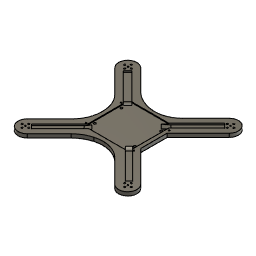
drone frame v1 (Autodesk Fusion 360 design; units mm, degrees)
Autodesk Fusion 360 part; units mm, degrees
note: some values were not read from the file. Chosen so that the rebuilt part matches the saved one: which face or edge a step refers to; which pieces of a blend or face edit are solid. Set by a fixed rule: which sketch regions a step uses.
sketch "Sketch1" plane through (0, 0, 0) normal (0, 1, 0) x (1, 0, 0)
  line L0 (0, 0) -> (-60, 0)
  line L1 (-60, 0) -> (-60, 60)
  line L2 (-60, 60) -> (0, 60)
  line L3 (0, 60) -> (0, 0)
  line L4 (5, -5) -> (-65, -5)
  line L5 (-65, -5) -> (-65, 65)
  line L6 (-65, 65) -> (5, 65)
  line L7 (5, 65) -> (5, -5)
  dimension "d1" = 60
  dimension "d2" = 60
  dimension "d4" = 5
  dimension "d5" = 5
  dimension "d6" = 5
  constraint horizontal L0
  constraint vertical L1
  constraint horizontal L2
  constraint vertical L3
  constraint coincident L0.start L3.end
  constraint horizontal L4
  constraint vertical L5
  constraint horizontal L6
  constraint vertical L7
  measures "d1" distance of L0.start L0.end
  measures "d2" distance of L0.start L2.end
  measures "d4" distance of L0 L4
  measures "d5" distance of L2 L6
  measures "d6" distance of L1 L5
sketch "Sketch2" plane through (0, 0, 0) normal (0, 1, 0) x (1, 0, 0)
  line L0 (-65.6777, 47.3223) -> (-48, 65)
  line L1 (-48, 65) -> (-90.4264, 107.4264)
  line L2 (-108.1041, 89.7487) -> (-65.6777, 47.3223)
  line L3 (-12.6777, 65.6777) -> (5, 48)
  line L4 (5, 48) -> (47.4264, 90.4264)
  line L5 (29.7487, 108.1041) -> (-12.6777, 65.6777)
  line L6 (-47.3223, -5.6777) -> (-65, 12)
  line L7 (-65, 12) -> (-107.4264, -30.4264)
  line L8 (-89.7487, -48.1041) -> (-47.3223, -5.6777)
  line L9 (-12.6777, -5.6777) -> (5, 12)
  line L10 (5, 12) -> (47.4264, -30.4264)
  line L11 (29.7487, -48.1041) -> (-12.6777, -5.6777)
  arc A0 (-90.4264, 107.4264) -> (-108.1041, 89.7487) centre (-99.2652, 98.5876) ccw
  arc A1 (47.4264, 90.4264) -> (29.7487, 108.1041) centre (38.5876, 99.2652) ccw
  arc A2 (29.7487, -48.1041) -> (47.4264, -30.4264) centre (38.5876, -39.2652) ccw
  arc A3 (-107.4264, -30.4264) -> (-89.7487, -48.1041) centre (-98.5876, -39.2652) ccw
  dimension "d7" = 60
  dimension "d8" = 60
  dimension "d9" = 60
  dimension "d10" = 60
  dimension "d11" = 25
  dimension "d12" = 25
  dimension "d13" = 25
  dimension "d14" = 25
  constraint perpendicular L0 L1
  constraint parallel L1 L2
  constraint perpendicular L3 L4
  constraint parallel L4 L5
  constraint perpendicular L6 L7
  constraint parallel L7 L8
  constraint perpendicular L9 L10
  constraint parallel L10 L11
  constraint tangent L2 A0
  constraint tangent L1 A0
  constraint tangent L11 A2
  constraint tangent L10 A2
  constraint tangent L8 A3
  measures "d7" distance of L0.start L2.start
  measures "d8" distance of L3.start L5.start
  measures "d9" distance of L6.start L8.start
  measures "d10" distance of L9.start L11.start
  measures "d11" distance of L7 L8
  measures "d12" distance of L1 L2
  measures "d13" distance of L4 L5
  measures "d14" distance of L10 L11
extrude "Extrude1" add sketch "Sketch1" sketch "Sketch2" along normal blind 10 contours L0 L1 L2 L3 | L4 L5 L6 L7 of sketch 2
sketch "Sketch4" plane through (0, 5, 0) normal (0, 1, 0) x (-1, 0, 0)
  line L0 (5, -55.7066) -> (55, -55.7066)
  line L1 (55, -55.7066) -> (55, -4.4949)
  line L2 (55, -4.4949) -> (5, -4.4949)
  line L3 (5, -4.4949) -> (5, -55.7066)
  line L4 (6, -7) -> (11, -7)
  line L5 (11, -7) -> (11, -54)
  line L6 (11, -54) -> (6, -54)
  line L7 (6, -54) -> (6, -7)
  constraint horizontal L4
  constraint vertical L5
  constraint horizontal L6
  constraint vertical L7
sketch "Sketch6" plane through (0, 10, 0) normal (0, 1, 0) x (-1, 0, 0)
  line L0 (48, 5) -> (12, 5)
  line L1 (12, 5) -> (12.6777, 5.6777)
  line L2 (12.6777, 5.6777) -> (-29.7487, 48.1041)
  arc A0 (-29.7487, 48.1041) -> (-47.4264, 30.4264) centre (-38.5876, 39.2652) ccw
  line L3 (-47.4264, 30.4264) -> (-5, -12)
  line L4 (-5, -12) -> (-5, -48)
  line L5 (-5, -48) -> (-47.4264, -90.4264)
  arc A1 (-47.4264, -90.4264) -> (-29.7487, -108.1041) centre (-38.5876, -99.2652) ccw
  line L6 (-29.7487, -108.1041) -> (12.6777, -65.6777)
  line L7 (12.6777, -65.6777) -> (12, -65)
  line L8 (12, -65) -> (48, -65)
  line L9 (48, -65) -> (90.4264, -107.4264)
  arc A2 (90.4264, -107.4264) -> (108.1041, -89.7487) centre (99.2652, -98.5876) ccw
  line L10 (108.1041, -89.7487) -> (65.6777, -47.3223)
  line L11 (65.6777, -47.3223) -> (65, -48)
  line L12 (65, -48) -> (65, -12)
  line L13 (65, -12) -> (107.4264, 30.4264)
  arc A3 (107.4264, 30.4264) -> (89.7487, 48.1041) centre (98.5876, 39.2652) ccw
  line L14 (89.7487, 48.1041) -> (47.3223, 5.6777)
  line L15 (47.3223, 5.6777) -> (48, 5)
  circle A4 centre (0, 0) radius 1.5
  line L16 (0, 0) -> (60, 0)
  line L17 (60, 0) -> (29.3601, 0)
  circle A5 centre (60, 0) radius 1.5
  line L18 (0, 0) -> (0, -61)
  circle A6 centre (0, -61) radius 1.5
  line L19 (0, -61) -> (60, -61)
  line L20 (60, -61) -> (60, -64)
  circle A7 centre (60, -61) radius 1.5
  line L21 (60, -61) -> (60, 0)
  dimension "d23" = 3
  dimension "d24" = 30.6399
  dimension "d25" = 3
  dimension "d26" = 3
  dimension "d27" = 3
  dimension "d28" = 3
  constraint coincident A4.centre L16.start
  constraint horizontal L16
  constraint coincident L16 L17.end
  constraint coincident L16.end L17.start
  constraint perpendicular L16 L18
  constraint coincident L18.end A6.centre
  constraint perpendicular L18 L19
  constraint perpendicular L19 L20
  constraint coincident L19.end L20.start
  constraint perpendicular L16 L21
  measures "d23" diameter of A4
  measures "d24" distance of L16.end L17.end
  measures "d25" diameter of A5
  measures "d26" diameter of A6
  measures "d27" distance of L19.end L20.end
  measures "d28" diameter of A7
extrude "Extrude5" cut sketch "Sketch6" against normal blind 2 contours A4 L16 L17 A5 L18 A6 L19 A7 L21
extrude "Extrude7" cut 1 faces at (-85.225, 10, 26.1768) along direction (0, -1, 0) blind 5
extrude "Extrude8" cut 1 faces at (-39.6726, 8, -40.2888) along direction (0, -1, 0) blind 2
extrude "Extrude9" cut 1 faces at (-39.6726, 6, -40.2888) along direction (0, -1, 0) blind 2
sketch "Sketch8" plane through (0, 5, 0) normal (0, 1, 0) x (-1, 0, 0)
  line L0 (60, -1.5) -> (60, -59.5)
  line L1 (58.5, -61) -> (1.5, -61)
  line L2 (0, -59.5) -> (0, -1.5)
  line L3 (1.5, 0) -> (58.5, 0)
  line L4 (48, 5) -> (12, 5)
  line L5 (12, 5) -> (12.6777, 5.6777)
  line L6 (12.6777, 5.6777) -> (-29.7487, 48.1041)
  arc A0 (-29.7487, 48.1041) -> (-47.4264, 30.4264) centre (-38.5876, 39.2652) ccw
  line L7 (-47.4264, 30.4264) -> (-5, -12)
  line L8 (-5, -12) -> (-5, -48)
  line L9 (-5, -48) -> (-47.4264, -90.4264)
  arc A1 (-47.4264, -90.4264) -> (-29.7487, -108.1041) centre (-38.5876, -99.2652) ccw
  line L10 (-29.7487, -108.1041) -> (12.6777, -65.6777)
  line L11 (12.6777, -65.6777) -> (12, -65)
  line L12 (12, -65) -> (48, -65)
  line L13 (48, -65) -> (90.4264, -107.4264)
  arc A2 (90.4264, -107.4264) -> (108.1041, -89.7487) centre (99.2652, -98.5876) ccw
  line L14 (108.1041, -89.7487) -> (65.6777, -47.3223)
  line L15 (65.6777, -47.3223) -> (65, -48)
  line L16 (65, -48) -> (65, -12)
  line L17 (65, -12) -> (107.4264, 30.4264)
  arc A3 (107.4264, 30.4264) -> (89.7487, 48.1041) centre (98.5876, 39.2652) ccw
  line L18 (89.7487, 48.1041) -> (47.3223, 5.6777)
  line L19 (47.3223, 5.6777) -> (48, 5)
  arc A4 (0, -1.5) -> (1.5, 0) centre (0, 0) ccw
  arc A5 (58.5, 0) -> (60, -1.5) centre (60, 0) ccw
  arc A6 (60, -59.5) -> (58.5, -61) centre (60, -61) ccw
  arc A7 (1.5, -61) -> (0, -59.5) centre (0, -61) ccw
sketch "Sketch9" plane through (0, 5, 0) normal (0, 1, 0) x (-1, 0, 0)
sketch "Sketch10" plane through (0, 5, 0) normal (0, 1, 0) x (-1, 0, 0)
  line L0 (-39.5, 38) -> (-37.6, 38)
  circle A0 centre (-38.55, 39.15) radius 1.5116
  constraint horizontal L0
sketch "Sketch14" plane through (-30.3388, 5, -30) normal (0, 1, 0) x (-1, 0, 0)
  circle A0 centre (-70, 70) radius 4.5
  circle A1 centre (-70, 70) radius 1
  line L0 (-70, 70) -> (-70, 65.5)
  circle A2 centre (-70, 65.5) radius 1.12
  line L1 (-70, 70) -> (-70, 74.5)
  circle A3 centre (-70, 74.5) radius 1.12
  line L2 (-70, 70) -> (-65.5, 70)
  circle A4 centre (-65.5, 70) radius 1.12
  line L3 (-70, 70) -> (-74.5, 70)
  circle A5 centre (-74.5, 70) radius 1.12
  circle A6 centre (-70, -65.5) radius 1.12
  circle A7 centre (-65.5, -70) radius 1.12
  circle A8 centre (-70, -70) radius 4.5
  circle A9 centre (-70, -70) radius 1
  circle A10 centre (-70, -74.5) radius 1.12
  line L4 (-70, -70) -> (-70, -74.5)
  line L5 (-70, -70) -> (-70, -65.5)
  line L6 (-70, -70) -> (-74.5, -70)
  line L7 (-70, -70) -> (-65.5, -70)
  circle A11 centre (-74.5, -70) radius 1.12
  circle A12 centre (65.5, -70) radius 1.12
  circle A13 centre (70, -65.5) radius 1.12
  circle A14 centre (70, -70) radius 4.5
  circle A15 centre (70, -70) radius 1
  circle A16 centre (74.5, -70) radius 1.12
  line L8 (70, -70) -> (74.5, -70)
  line L9 (70, -70) -> (65.5, -70)
  line L10 (70, -70) -> (70, -74.5)
  line L11 (70, -70) -> (70, -65.5)
  circle A17 centre (70, -74.5) radius 1.12
  circle A18 centre (70, 65.5) radius 1.12
  circle A19 centre (65.5, 70) radius 1.12
  circle A20 centre (70, 70) radius 4.5
  circle A21 centre (70, 70) radius 1
  circle A22 centre (70, 74.5) radius 1.12
  line L12 (70, 70) -> (70, 74.5)
  line L13 (70, 70) -> (70, 65.5)
  line L14 (70, 70) -> (74.5, 70)
  line L15 (70, 70) -> (65.5, 70)
  circle A23 centre (74.5, 70) radius 1.12
  dimension "d46" = 9
  dimension "d47" = 2
  dimension "d48" = 4.5
  dimension "d49" = 2.24
  dimension "d50" = 4.5
  dimension "d51" = 2.24
  dimension "d52" = 4.5
  dimension "d53" = 2.24
  dimension "d54" = 4.5
  dimension "d55" = 2.24
  dimension "d57" = 360
  constraint concentric A0 A1
  constraint coincident A0.centre A1.centre
  constraint vertical L0
  constraint coincident L0.end A2.centre
  constraint parallel L0 L1
  constraint coincident L1.end A3.centre
  constraint perpendicular L0 L2
  constraint coincident L2.end A4.centre
  constraint perpendicular L0 L3
  constraint coincident L3.end A5.centre
  measures "d46" diameter of A0
  measures "d47" diameter of A1
  measures "d48" distance of A0.centre L0.end
  measures "d49" diameter of A2
  measures "d50" distance of A0.centre L1.end
  measures "d51" diameter of A3
  measures "d52" distance of A0.centre L2.end
  measures "d53" diameter of A4
  measures "d54" distance of A0.centre L3.end
  measures "d55" diameter of A5
extrude "Extrude11" cut sketch "Sketch14" against normal blind 80 contours A0 L2 A4 | A0 A4 | A0 L2 A4 | A0 L1 A3 | A0 A3 | A0 A2 | A0 L0 A2 | A1 L1 L2 | A1 L0 L2 | A0 L1 A3 | A0 L0 A2 | A1 L1 L3 | A1 L0 L3 | A0 L3 A5 | A0 A5 | A0 L3 A5 | A6 A8 | A6 A8 L5 | A6 A8 L5 | A8 L6 A11 | A8 A11 | A7 A8 L7 | A7 A8 | A9 L5 L6 | A9 L5 L7 | A8 L6 A11 | A7 A8 L7 | A9 L4 L7 | A9 L4 L6 | A8 A10 L4 | A8 A10 | A8 A10 L4 | A12 A14 L9 | A12 A14 L9 | A12 A14 | A15 L9 L10 | A15 L9 L11 | A13 A14 L11 | A13 A14 | A14 L10 A17 | A14 A17 | A15 L8 L11 | A15 L8 L10 | A13 A14 L11 | A14 L10 A17 | A14 A16 L8 | A14 A16 L8 | A14 A16 | A18 A20 | A18 A20 L13 | A18 A20 L13 | A20 L14 A23 | A20 A23 | A19 A20 L15 | A19 A20 | A21 L13 L14 | A21 L13 L15 | A20 L14 A23 | A19 A20 L15 | A21 L12 L15 | A21 L12 L14 | A20 A22 | A20 A22 L12 | A20 A22 L12
sketch "Sketch15" plane through (0, 5, 0) normal (0, 1, 0) x (-1, 0, 0)
  circle A0 centre (-35.1612, 40) radius 1.12
  circle A1 centre (-35.1612, -100) radius 1.12
  circle A2 centre (100.3388, -95.5) radius 1.12
  circle A3 centre (100.3388, -104.5) radius 1.12
  circle A4 centre (100.3388, 44.5) radius 1.12
  circle A5 centre (100.3388, 40) radius 1
  circle A6 centre (95.8388, -100) radius 1.12
  circle A7 centre (-39.6612, -104.5) radius 1.12
  circle A8 centre (-39.6612, -95.5) radius 1.12
  circle A9 centre (-39.6612, 44.5) radius 1.12
  circle A10 centre (-39.6612, 40) radius 1
  circle A11 centre (-39.6612, -100) radius 1
  circle A12 centre (104.8388, -100) radius 1.12
  circle A13 centre (95.8388, 40) radius 1.12
  circle A14 centre (104.8388, 40) radius 1.12
  circle A15 centre (100.3388, 35.5) radius 1.12
  circle A16 centre (100.3388, -100) radius 1
  circle A17 centre (-44.1612, -100) radius 1.12
  circle A18 centre (-39.6612, 35.5) radius 1.12
  circle A19 centre (-44.1612, 40) radius 1.12
  arc A20 (0, -1.5) -> (1.5, 0) centre (0, 0) ccw
  line L0 (1.5, 0) -> (58.5, 0)
  arc A21 (58.5, 0) -> (60, -1.5) centre (60, 0) ccw
  line L1 (60, -1.5) -> (60, -59.5)
  arc A22 (60, -59.5) -> (58.5, -61) centre (60, -61) ccw
  line L2 (58.5, -61) -> (1.5, -61)
  arc A23 (1.5, -61) -> (0, -59.5) centre (0, -61) ccw
  line L3 (0, -59.5) -> (0, -1.5)
  line L4 (48, 5) -> (12, 5)
  line L5 (12, 5) -> (12.6777, 5.6777)
  line L6 (12.6777, 5.6777) -> (-29.7487, 48.1041)
  arc A24 (-29.7487, 48.1041) -> (-47.4264, 30.4264) centre (-38.5876, 39.2652) ccw
  line L7 (-47.4264, 30.4264) -> (-5, -12)
  line L8 (-5, -12) -> (-5, -48)
  line L9 (-5, -48) -> (-47.4264, -90.4264)
  arc A25 (-47.4264, -90.4264) -> (-29.7487, -108.1041) centre (-38.5876, -99.2652) ccw
  line L10 (-29.7487, -108.1041) -> (12.6777, -65.6777)
  line L11 (12.6777, -65.6777) -> (12, -65)
  line L12 (12, -65) -> (48, -65)
  line L13 (48, -65) -> (90.4264, -107.4264)
  arc A26 (90.4264, -107.4264) -> (108.1041, -89.7487) centre (99.2652, -98.5876) ccw
  line L14 (108.1041, -89.7487) -> (65.6777, -47.3223)
  line L15 (65.6777, -47.3223) -> (65, -48)
  line L16 (65, -48) -> (65, -12)
  line L17 (65, -12) -> (107.4264, 30.4264)
  arc A27 (107.4264, 30.4264) -> (89.7487, 48.1041) centre (98.5876, 39.2652) ccw
  line L18 (89.7487, 48.1041) -> (47.3223, 5.6777)
  line L19 (47.3223, 5.6777) -> (48, 5)
  line L20 (-38, 32) -> (-33, 37)
  line L21 (-33, 37) -> (9.0734, -5.0734)
  line L22 (9.0734, -5.0734) -> (4.0734, -10.0734)
  line L23 (4.0734, -10.0734) -> (-38, 32)
  line L24 (93, 39) -> (98.4268, 33.5732)
  line L25 (98.4268, 33.5732) -> (57.2172, -7.6363)
  line L26 (57.2172, -7.6363) -> (51.7904, -2.2096)
  line L27 (51.7904, -2.2096) -> (93, 39)
  line L28 (98.7842, -91.9686) -> (92.911, -97.8418)
  line L29 (92.911, -97.8418) -> (52.9278, -57.8585)
  line L30 (52.9278, -57.8585) -> (58.801, -51.9853)
  line L31 (58.801, -51.9853) -> (98.7842, -91.9686)
  line L32 (-32.4189, -99.1776) -> (-38.1738, -93.4227)
  line L33 (-38.1738, -93.4227) -> (5.1244, -50.1244)
  line L34 (5.1244, -50.1244) -> (10.8793, -55.8793)
  line L35 (10.8793, -55.8793) -> (-32.4189, -99.1776)
  constraint perpendicular L20 L21
  constraint parallel L20 L22
  constraint parallel L21 L23
  constraint perpendicular L6 L20
  constraint perpendicular L24 L25
  constraint parallel L24 L26
  constraint parallel L25 L27
  constraint perpendicular L18 L24
  constraint perpendicular L28 L29
  constraint parallel L28 L30
  constraint parallel L29 L31
  constraint perpendicular L14 L28
  constraint perpendicular L32 L33
  constraint parallel L32 L34
  constraint parallel L33 L35
  constraint perpendicular L10 L32
extrude "Extrude12" cut sketch "Sketch15" against normal blind 2 contours A20 L0 L3 L20 L21 L23 | A20 L0 L3 L21 L22 L23 | L2 A23 L3 L33 L34 L35 | L2 A23 L3 L32 L33 L35 | L0 A21 L1 L24 L25 L27 | L0 A21 L1 L25 L26 L27 | L1 A22 L2 L29 L30 L31 | L1 A22 L2 L28 L29 L31
sketch "ELECTRONICS iNSIDE" plane through (0, 4, 0) normal (0, 1, 0) x (-1, 0, 0)
  line L0 (60, -4.8535) -> (57.2172, -7.6363)
  line L1 (57.2172, -7.6363) -> (51.7904, -2.2096)
  line L2 (51.7904, -2.2096) -> (54, 0)
  line L3 (54, 0) -> (4, 0)
  line L4 (4, 0) -> (9.0734, -5.0734)
  line L5 (9.0734, -5.0734) -> (4.0734, -10.0734)
  line L6 (4.0734, -10.0734) -> (0, -6)
  line L7 (0, -6) -> (0, -55.2489)
  line L8 (0, -55.2489) -> (5.1244, -50.1244)
  line L9 (5.1244, -50.1244) -> (10.8793, -55.8793)
  line L10 (10.8793, -55.8793) -> (5.7586, -61)
  line L11 (5.7586, -61) -> (56.0693, -61)
  line L12 (56.0693, -61) -> (52.9278, -57.8585)
  line L13 (52.9278, -57.8585) -> (58.801, -51.9853)
  line L14 (58.801, -51.9853) -> (60, -53.1843)
  line L15 (60, -53.1843) -> (60, -4.8535)
  circle A0 centre (2.5341, -47.5622) radius 1.5
  line L16 (2.5341, -47.5622) -> (57, -47.5622)
  line L17 (57, -47.5622) -> (57, -11.3447)
  line L18 (57, -11.3447) -> (2.5341, -11.3447)
  line L19 (2.5341, -11.3447) -> (2.5341, -47.5622)
  circle A1 centre (57, -47.5622) radius 1.5
  circle A2 centre (57, -11.3447) radius 1.5
  circle A3 centre (2.5341, -11.3447) radius 1.5
  dimension "d62" = 3
  dimension "d63" = 3
  dimension "d64" = 3
  dimension "d65" = 3
  constraint horizontal L16
  constraint vertical L17
  constraint horizontal L18
  constraint vertical L19
  constraint coincident A0.centre L16.start
  constraint coincident L16.end L17.start
  constraint coincident L17.end L18.start
  constraint coincident L18.end L19.start
  measures "d62" diameter of A0
  measures "d63" diameter of A1
  measures "d64" diameter of A2
  measures "d65" diameter of A3
extrude "Extrude13" cut sketch "ELECTRONICS iNSIDE" against normal blind 30 contours A0 L16 L19 | A0 L16 L19 | L16 L17 A1 | L16 L17 A1 | L18 L19 A3 | L18 L19 A3 | L17 L18 A2 | L17 L18 A2
sketch "OUTER MINI PC" plane through (0, 5, 0) normal (0, 1, 0) x (-1, 0, 0)
  line L0 (98.4268, 33.5732) -> (60, -4.8535)
  line L1 (60, -4.8535) -> (60, -53.1843)
  line L2 (60, -53.1843) -> (98.7842, -91.9686)
  line L3 (98.7842, -91.9686) -> (92.911, -97.8418)
  line L4 (92.911, -97.8418) -> (56.0693, -61)
  line L5 (56.0693, -61) -> (5.7586, -61)
  line L6 (5.7586, -61) -> (-32.4189, -99.1776)
  line L7 (-32.4189, -99.1776) -> (-38.1738, -93.4227)
  line L8 (-38.1738, -93.4227) -> (0, -55.2489)
  line L9 (0, -55.2489) -> (0, -6)
  line L10 (0, -6) -> (-38, 32)
  line L11 (-38, 32) -> (-33, 37)
  line L12 (-33, 37) -> (4, 0)
  line L13 (4, 0) -> (54, 0)
  line L14 (54, 0) -> (93, 39)
  line L15 (93, 39) -> (98.4268, 33.5732)
  circle A0 centre (-35.1612, 40) radius 1.12
  circle A1 centre (-35.1612, -100) radius 1.12
  circle A2 centre (100.3388, -95.5) radius 1.12
  circle A3 centre (100.3388, -104.5) radius 1.12
  circle A4 centre (100.3388, 44.5) radius 1.12
  circle A5 centre (100.3388, 40) radius 1
  circle A6 centre (95.8388, -100) radius 1.12
  circle A7 centre (-39.6612, -104.5) radius 1.12
  circle A8 centre (-39.6612, -95.5) radius 1.12
  circle A9 centre (-39.6612, 44.5) radius 1.12
  circle A10 centre (-39.6612, 40) radius 1
  circle A11 centre (-39.6612, -100) radius 1
  circle A12 centre (104.8388, -100) radius 1.12
  circle A13 centre (95.8388, 40) radius 1.12
  circle A14 centre (104.8388, 40) radius 1.12
  circle A15 centre (100.3388, 35.5) radius 1.12
  circle A16 centre (100.3388, -100) radius 1
  circle A17 centre (-44.1612, -100) radius 1.12
  circle A18 centre (-39.6612, 35.5) radius 1.12
  circle A19 centre (-44.1612, 40) radius 1.12
  line L16 (48, 5) -> (12, 5)
  line L17 (12, 5) -> (12.6777, 5.6777)
  line L18 (12.6777, 5.6777) -> (-29.7487, 48.1041)
  arc A20 (-29.7487, 48.1041) -> (-47.4264, 30.4264) centre (-38.5876, 39.2652) ccw
  line L19 (-47.4264, 30.4264) -> (-5, -12)
  line L20 (-5, -12) -> (-5, -48)
  line L21 (-5, -48) -> (-47.4264, -90.4264)
  arc A21 (-47.4264, -90.4264) -> (-29.7487, -108.1041) centre (-38.5876, -99.2652) ccw
  line L22 (-29.7487, -108.1041) -> (12.6777, -65.6777)
  line L23 (12.6777, -65.6777) -> (12, -65)
  line L24 (12, -65) -> (48, -65)
  line L25 (48, -65) -> (90.4264, -107.4264)
  arc A22 (90.4264, -107.4264) -> (108.1041, -89.7487) centre (99.2652, -98.5876) ccw
  line L26 (108.1041, -89.7487) -> (65.6777, -47.3223)
  line L27 (65.6777, -47.3223) -> (65, -48)
  line L28 (65, -48) -> (65, -12)
  line L29 (65, -12) -> (107.4264, 30.4264)
  arc A23 (107.4264, 30.4264) -> (89.7487, 48.1041) centre (98.5876, 39.2652) ccw
  line L30 (89.7487, 48.1041) -> (47.3223, 5.6777)
  line L31 (47.3223, 5.6777) -> (48, 5)
  circle A24 centre (62.5, -4.7474) radius 1
  line L32 (62.5, -4.7474) -> (62.5, -52.8012)
  line L33 (62.5, -52.8012) -> (65, -52.8012)
  circle A25 centre (62.5, -52.8012) radius 1
  line L34 (62.5, -4.7474) -> (-2.9935, -4.7474)
  line L35 (-2.9935, -4.7474) -> (-3.0065, -7.1072)
  circle A26 centre (-2.9935, -4.7474) radius 1
  line L36 (62.5, -52.8012) -> (-3, -52.8012)
  line L37 (-3, -52.8012) -> (-3, -5.9273)
  line L38 (-2.9935, -4.7474) -> (-3.5, -4.7474)
  circle A27 centre (-3, -52.8012) radius 1
  dimension "d68" = 2
  dimension "d69" = 2.5
  dimension "d70" = 2
  dimension "d71" = 2.3599
  dimension "d72" = 2
  dimension "d73" = 2
  constraint coincident A24.centre L32.start
  constraint parallel L1 L32
  constraint perpendicular L32 L33
  constraint coincident L32.end L33.start
  constraint perpendicular L9 L34
  constraint coincident L34.end L35.start
  constraint perpendicular L9 L36
  constraint midpoint L35 L37.end
  constraint perpendicular L34 L37
  constraint coincident L34 L38.end
  constraint coincident L36.end L37.start
  measures "d68" diameter of A24
  measures "d69" distance of L32.end L33.end
  measures "d70" diameter of A25
  measures "d71" distance of L34.end L35.end
  measures "d72" diameter of A26
  measures "d73" diameter of A27
extrude "Extrude14" cut sketch "OUTER MINI PC" against normal blind 29 contours A24 L32 L34 | A24 L32 L34 | L34 L35 A26 | L34 L35 A26 | L33 A25 L36 | L32 A25 L36 | L32 L33 A25 | L36 L37 A27 | L36 L37 A27
fillet "Fillet1" radius 10.25 1 edges at (-47.3223, 2.5, 5.6777)
fillet "Fillet2" radius 45 1 edges at (-48, 2.5, 5)
fillet "Fillet3" radius 32 1 edges at (-12.6777, 2.5, 5.6777)
fillet "Fillet4" radius 39.5 1 edges at (-12, 2.5, 5)
fillet "Fillet5" radius 48 1 edges at (-48, 2.5, -65)
fillet "Fillet6" radius 10.7 1 edges at (-12.6777, 2.5, -65.6777)
fillet "Fillet7" radius 37.5 1 edges at (-12, 2.5, -65)
fillet "Fillet8" radius 18 1 edges at (-65.6777, 2.5, -47.3223)
fillet "Fillet9" radius 38.5 1 edges at (-65, 2.5, -48)
fillet "Fillet10" radius 38.5 1 edges at (-65, 2.5, -12)
fillet "Fillet11" radius 43.5 1 edges at (-8.0019, 3, -53.0019)
fillet "Fillet12" radius 29 1 edges at (-55.8644, 3, -54.9219)
fillet "Fillet13" radius 29 1 edges at (-54.5038, 3, -4.923)
fillet "Fillet14" radius 22 1 edges at (-6.5734, 3, -7.5734)
